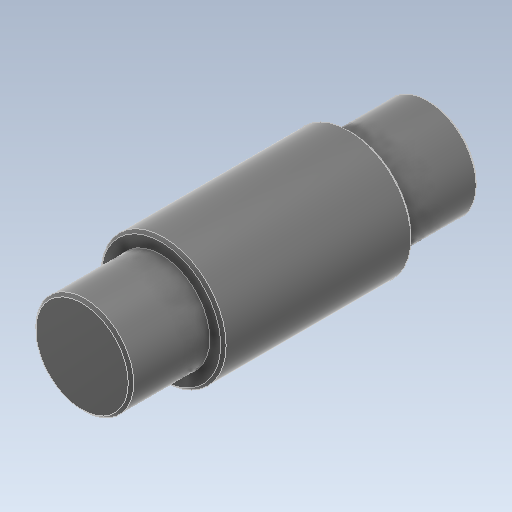
# Autodesk Inventor part: Peça13
Saved by Autodesk Inventor 2021 (Build 250183000, 183)
## iProperties
Category: 41
Created: 2021-07-17
Part Number: Peça13
Material: Liga de aço
Document SubType Name: Modeling
Designer: Giovanni
Density: 7.73 g/cm^3
Appearance: Liso - Preto
User Status: 1:2
Author: Giovanni
Keywords: 8
Autodesk Inventor part; units mm, degrees
ref_plane "YZ Plane" through (0, 0, 0) normal (1, 0, 0) x (0, 1, 0)
ref_plane "XZ Plane" through (0, 0, 0) normal (0, 1, 0) x (-1, 0, 0)
ref_plane "XY Plane" through (0, 0, 0) normal (0, 0, 1) x (1, 0, 0)
sketch "Esboço1" plane through (0, 0, 0) normal (0, 0, 1) x (-1, 0, 0)
  circle A0 centre (0, 0) radius 23
  dimension "d0" = 46
  constraints: 1 centre point, 1 coincident
  measures "d0" diameter of A0
extrude "Extrusão1" add sketch "Esboço1" along normal mid plane 70
sketch "Esboço2" plane through (0, 0, -35) normal (0, 0, -1) x (1, 0, 0)
  circle A0 centre (0, 0) radius 18
  dimension "d3" = 36
  constraints: 1 centre point, 1 coincident
  measures "d3" diameter of A0
extrude "Extrusão2" add sketch "Esboço2" along normal blind 29
sketch "Esboço3" plane through (0, 0, 35) normal (0, 0, 1) x (1, 0, 0)
  circle A0 centre (0, 0) radius 18
  dimension "d6" = 36
  constraints: 1 centre point, 1 coincident
  measures "d6" diameter of A0
extrude "Extrusão3" add sketch "Esboço3" along normal blind 29
chamfer "Chanfro1" distance 1 angle 45 1 edges at (-18, 0, -64)
chamfer "Chanfro2" distance 1 angle 45 3 edges at (23, 0, -35) (23, 0, 35) (-18, 0, 64)
